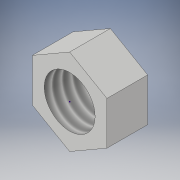
# Autodesk Inventor part: .125nut
Saved by Autodesk Inventor 2017 (Build 210142000, 142)
## iProperties
Created: 2017-04-26
Part Number: .125nut
Material: Generic
Document SubType Name: Modeling
Designer: User
Density: 1 g/cm^3
Appearance: Default
Author: User
Autodesk Inventor part; units mm, degrees
ref_plane "YZ Plane" through (0, 0, 0) normal (1, 0, 0) x (0, 1, 0)
ref_plane "XZ Plane" through (0, 0, 0) normal (0, 1, 0) x (-1, 0, 0)
ref_plane "XY Plane" through (0, 0, 0) normal (0, 0, 1) x (1, 0, 0)
sketch "Sketch1" plane through (0, 0, 0) normal (0, 0, 1) x (1, 0, 0)
  circle A0 centre (0, 0) radius 1.5875
  line L0 (0, 2.6857) -> (2.3259, 1.3428)
  line L1 (2.3259, 1.3428) -> (2.3259, -1.3428)
  line L2 (2.3259, -1.3428) -> (0, -2.6857)
  line L3 (0, -2.6857) -> (-2.3259, -1.3428)
  line L4 (-2.3259, -1.3428) -> (-2.3259, 1.3428)
  line L5 (-2.3259, 1.3428) -> (0, 2.6857)
  dimension "d0" = 3.175
  constraints: 12 end point, 2 coincident, 1 centre point, 13 other
  measures "d0" diameter of A0
extrude "Extrusion1" add sketch "Sketch1" along normal blind 2.54
sketch "Sketch2" plane through (0, 0, 2.54) normal (0, 0, 1) x (1, 0, 0)
  point P0 (0, 0)
  point P1 (0, 0)
  constraints: 1 coincident
thread "Thread1" size "5-40 UNC" class "2B" standard "ANSI Unified Screw Threads" full length
body "Solid1"
